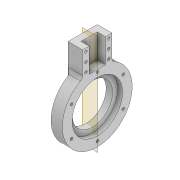
# Autodesk Inventor part: Bearing_housing
Saved by Autodesk Inventor 2022 (Build 260153000, 153)
## iProperties
Created: 2022-07-04
Part Number: Bearing_housing
Material: Generic
Document SubType Name: Modeling
Designer: dell
Density: 1 g/cm^3
Appearance: Default
Author: dell
Autodesk Inventor part; units mm, degrees
ref_plane "YZ Plane" through (0, 0, 0) normal (1, 0, 0) x (0, 1, 0)
sketch "Sketch1" plane through (0, 0, 0) normal (1, 0, 0) x (0, 1, 0)
  circle A0 centre (0, 0) radius 31.25
  circle A1 centre (0, 0) radius 43.25
  circle A2 centre (0, 0) radius 25
  dimension "d0" = 62.5
  dimension "d1" = 12
  dimension "d2" = 50
  constraints: 3 centre point, 2 coincident
  measures "d0" diameter of A0
  measures "d1" radial gap between concentric circles of A0 A1
  measures "d2" diameter of A2
extrude "Extrusion1" add sketch "Sketch1" along normal blind 8 contours A0 | A1
sketch "Sketch2" plane through (8, 0, 0) normal (1, 0, 0) x (0, 0, -1)
  circle A0 centre (0, 0) radius 31.25
  circle A1 centre (0, 0) radius 43.25 projected
  circle A2 centre (0, 0) radius 25 projected
  dimension "d5" = 62.5
  constraints: 1 centre point, 1 coincident
  measures "d5" diameter of A0
extrude "Extrusion2" add sketch "Sketch2" along normal blind 6 contours A1
sketch "Sketch3" plane through (14, 0, 0) normal (1, 0, 0) x (0, 0, -1)
  circle A0 centre (0, 37) radius 1.6
  point P0 (0, 0)
  dimension "d8" = 3.2
  dimension "d9" = 37
  constraints: 1 centre point
  measures "d8" diameter of A0
  measures "d9" distance of point (0, 0) A0.centre
extrude "Extrusion3" cut sketch "Sketch3" against normal blind 100
pattern_circular "Circular Pattern1" count 6 over 360 about axis through (-10, 0, 0) along (1, 0, 0) of "Extrusion3"
ref_plane "Work Plane1" through (0, 40, 0) normal (0, 1, 0) x (-1, 0, 0)
sketch "Sketch4" plane through (0, 40, 0) normal (0, 1, 0) x (-1, 0, 0)
  line L0 (-14, 43.25) -> (-14, -43.25) projected
  line L1 (-14, 10.1) -> (-3.9, 10.1)
  line L2 (-3.9, 10.1) -> (-3.9, -10.1)
  line L3 (-3.9, -10.1) -> (-14, -10.1)
  line L4 (-14, -10.1) -> (-14, 10.1)
  line L5 (-14, 18.1) -> (0, 18.1)
  line L6 (0, 18.1) -> (0, -18.1)
  line L7 (0, -18.1) -> (-14, -18.1)
  line L8 (0, 43.25) -> (0, -43.25) projected
  point P0 (0, 0)
  point P1 (0, 0)
  point P2 (-14, -10.1)
  dimension "d16" = 10.1
  dimension "d17" = 20.2
  dimension "d18" = 10.1
  dimension "d20" = 8
  dimension "d21" = 8
  constraints: 14 end point, 3 perpendicular, 3 point on line, 2 horizontal, 2 midpoint, 2 parallel
  measures "d16" distance of L2.end L3.end
  measures "d17" distance between parallel lines of L1 L3
  measures "d18" distance from line of point (0, 0) L1
  measures "d20" distance between parallel lines of L3 L7
  measures "d21" distance between parallel lines of L5 L1
extrude "Extrusion4" cut sketch "Sketch4" along normal blind 100
extrude "Extrusion5" add sketch "Sketch4" along normal blind 30 contours L5 L6 L7 L0 L3 L2 L1
fillet "Fillet1" radius 5 2 edges at (7, 40, 16.4488) (7, 40, -16.4488)
sketch "Sketch7" plane through (0, 0, 0) normal (-1, 0, 0) x (0, 0, 1)
  arc A0 (18.1, 40) -> (19.9211, 38.389) centre (22.2241, 42.827) ccw projected
  line L0 (18.1, 40) -> (18.1, 17.245)
  circle A1 centre (0, 0) radius 25 projected
  arc A2 (-19.9211, 38.389) -> (-18.1, 40) centre (-22.2241, 42.827) ccw projected
  line L1 (-18.1, 40) -> (-18.1, 17.2187)
  line L2 (-18.1, 70) -> (18.1, 70) projected
  line L3 (-18.1, 40) -> (18.1, 40)
  line L4 (18.1, 40) -> (18.1, 70)
  line L5 (18.1, 70) -> (-18.1, 70)
  line L6 (-18.1, 70) -> (-18.1, 40)
  circle A3 centre (0, 0) radius 34
  point P0 (-18.1, 28.7818)
  point P1 (18.1, 28.7818)
  dimension "d34" = 9
  constraints: 12 end point, 2 parallel, 2 vertical, 1 centre point, 1 horizontal, 1 perpendicular, 2 other
extrude "Extrusion6" add sketch "Sketch7" along normal blind 4 contours L0 A3 L1 L3 | L3 L6 L2 L4
fillet "Fillet2" radius 5 4 edges at (0, 34.3909, -18.1) (0, 34.3909, 18.1) (7, 40, 18.1) (7, 40, -18.1)
sketch "Sketch6" plane through (14, 0, 0) normal (1, 0, 0) x (0, 0, -1)
  circle A0 centre (-14.1, 44) radius 1.6
  circle A1 centre (-14.1, 55) radius 1.6
  circle A2 centre (-14.1, 66) radius 1.6
  line L0 (-60.55, 40) -> (60.55, 40) projected
  line L1 (-18.1, 70) -> (-10.1, 70) projected
  line L2 (-18.1, 40) -> (-18.1, 70) projected
  point P0 (0, 0)
  dimension "d27" = 3.2
  dimension "d28" = 3.2
  dimension "d29" = 3.2
  dimension "d30" = 4
  dimension "d31" = 4
  dimension "d32" = 15
  dimension "d33" = 4
  constraints: 3 centre point, 2 vertical alignment
  measures "d27" diameter of A0
  measures "d28" diameter of A1
  measures "d29" diameter of A2
  measures "d30" distance from line of L0 A0.centre
  measures "d31" distance from line of L1 A2.centre
  measures "d32" distance from line of L0 A1.centre
  measures "d33" distance from line of L2 A0.centre
extrude "Extrusion7" cut sketch "Sketch6" against normal blind 100
mirror "Mirror1" about plane through (0, 0, 0) normal (0, 0, 1) of "Extrusion7"
equation "\"d18\" = 0.5 * d17"
body "Solid1"
